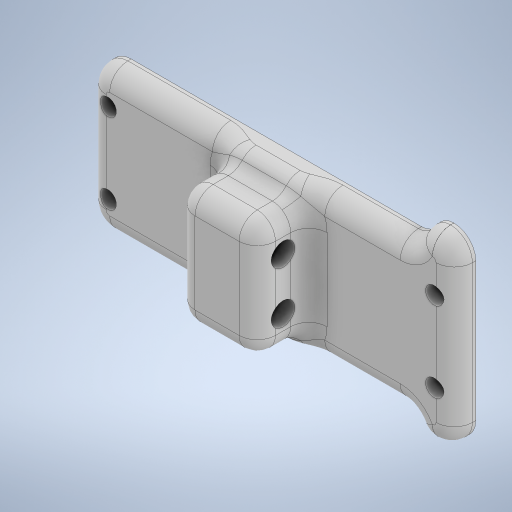
# Autodesk Inventor part: connecting plate servo flat v3
Saved by Autodesk Inventor 2024 (Build 280153000, 153)
## iProperties
Created: 2023-09-15
Part Number: connecting plate servo flat v3
Material: Generic
Document SubType Name: Modeling
Designer: chris
Density: 1 g/cm^3
Appearance: Default
Author: chris
Autodesk Inventor part; units mm, degrees
ref_plane "YZ Plane" through (0, 0, 0) normal (1, 0, 0) x (0, 1, 0)
ref_plane "XZ Plane" through (0, 0, 0) normal (0, 1, 0) x (-1, 0, 0)
ref_plane "XY Plane" through (0, 0, 0) normal (0, 0, 1) x (1, 0, 0)
sketch "Sketch1" plane through (0, 0, 0) normal (0, 0, 1) x (1, 0, 0)
  circle A0 centre (-10.2325, -6.35) radius 2
  circle A1 centre (-10.2325, 6.35) radius 2
  circle A2 centre (10.0875, 6.35) radius 2
  circle A3 centre (10.0875, -6.35) radius 2
  line L0 (-15.3125, 10.2775) -> (10.2325, 10.2775)
  line L1 (10.2325, 10.2775) -> (15.3125, 10.2775)
  line L2 (15.3125, 10.2775) -> (15.3125, -10.2775)
  line L3 (-15.3125, 10.2775) -> (-15.3125, -10.2775)
  line L4 (-15.3125, -10.2775) -> (15.3125, -10.2775)
  line L5 (0, -10.2775) -> (0, 10.2775)
  line L6 (-15.3125, 0) -> (0, 0)
  point P0 (0, 0)
  dimension "d1" = 5.08
  constraints: 14 end point, 4 centre point, 4 perpendicular, 3 midpoint, 1 point on line
  measures "d1" distance of L0.end L1.end
extrude "Extrusion1" add sketch "Sketch1" along normal blind 3.81 contours A0 | A1 | A2 | A3 | L0 L5 L6 L3 | L0 L1 L2 L4 L5 | L6 L5 L4 L3
sketch "Sketch2" plane through (0, 0, 3.81) normal (0, 0, 1) x (1, 0, 0)
  line L0 (-15.3125, -10.2775) -> (15.3125, -10.2775) projected
  line L1 (15.3125, -10.2775) -> (15.3125, 10.2775) projected
  line L2 (15.3125, 10.2775) -> (-15.3125, 10.2775) projected
  line L3 (-15.3125, 10.2775) -> (-15.3125, -10.2775) projected
  point P0 (0, 0)
extrude "Extrusion2" add sketch "Sketch2" along normal blind 1.5875
sketch "Sketch3" plane through (0, 0, 5.3975) normal (0, 0, 1) x (1, 0, 0)
  circle A0 centre (-10.2325, -6.35) radius 2 projected
  circle A1 centre (10.0875, -6.35) radius 2 projected
  circle A2 centre (10.0875, 6.35) radius 2 projected
  circle A3 centre (-10.2325, 6.35) radius 2 projected
  line L0 (-15.3125, -10.2775) -> (15.3125, -10.2775) projected
  line L1 (10.0875, -10.2775) -> (10.0875, 10.2775)
  line L2 (15.3125, 10.2775) -> (-15.3125, 10.2775) projected
  line L3 (-10.2325, -10.2775) -> (-10.2325, 10.2775)
  line L4 (-10.2325, 10.2775) -> (10.0875, 10.2775)
  line L5 (10.0875, -10.2775) -> (-10.2325, -10.2775)
  line L6 (15.3125, -10.2775) -> (15.3125, 10.2775) projected
  point P0 (0, 0)
  constraints: 8 end point, 2 point on line, 2 vertical, 1 parallel, 1 perpendicular
extrude "Extrusion3" add sketch "Sketch3" along normal blind 8.9916 contours A0 L3 | A0 L3 A3 L2 L1 A2 A1 L0 | L3 A3 | A1 L1 | L1 A2 picked at (-9.5825, -6.2017) picked at (-9.5825, 6.4983) picked at (9.4642, -6.5864) picked at (9.4642, 6.1136)
sketch "Sketch4" plane through (-10.2325, -10.2775, 5.3975) normal (-1, 0, 0) x (0, 0, 1)
  line L0 (8.9916, 20.555) -> (8.9916, 0) projected
  line L1 (8.9916, 10.2775) -> (0, 10.2775)
  line L2 (0, 0) -> (0, 20.555) projected
  line L3 (4.4958, 10.2775) -> (4.4958, 5.7817)
  line L4 (4.4958, 10.2775) -> (4.4958, 14.7733)
  circle A0 centre (4.4958, 5.7817) radius 2
  circle A1 centre (4.4958, 14.7733) radius 2
  point P0 (-5.3975, 10.2775)
  dimension "d8" = 4.4958
  dimension "d9" = 4.4958
  dimension "d10" = 4
  dimension "d11" = 4
  constraints: 6 end point, 3 midpoint, 2 centre point, 2 coincident, 2 vertical
  measures "d8" distance of L3.start L3.end
  measures "d9" distance of L3.start L4.end
  measures "d10" diameter of A0
  measures "d11" diameter of A1
extrude "Extrusion4" cut sketch "Sketch4" against normal through all
sketch "Sketch7" plane through (10.0875, -10.2775, 5.3975) normal (1, 0, 0) x (0, 0, -1)
  line L0 (0, 20.555) -> (0, 0) projected
  line L1 (0, 20.555) -> (-8.9916, 20.555) projected
  line L2 (-8.9916, 0) -> (-8.9916, 20.555) projected
  line L3 (0, 0) -> (-8.9916, 0) projected
  circle A0 centre (-4.4958, 14.7733) radius 2 projected
  circle A1 centre (-4.4958, 5.7817) radius 2 projected
  point P0 (5.3975, 10.2775)
extrude "Extrusion7" cut sketch "Sketch7" against normal blind 6.289 contours L0 L3 L2 L1 | A0 | A1
fillet "Fillet5" radius 3.175 8 edges at (-15.3125, 10.2775, 2.6987) (-15.3125, -10.2775, 2.6987) (15.3125, 10.2775, 2.6987) (15.3125, -10.2775, 2.6987) (3.7984, 10.2775, 9.8933) (-10.2325, 10.2775, 9.8933) (3.7984, -10.2775, 9.8933) (-10.2325, -10.2775, 9.8933)
sketch "Sketch9" plane through (0, 0, 0) normal (0, 0, -1) x (-1, 0, 0)
  line L0 (-34.8064, -15.875) -> (-34.8064, 15.875)
  line L1 (-27.8064, -15.875) -> (-34.8064, -15.875)
  line L2 (-27.8064, -12.5) -> (-27.8064, -15.875)
  line L3 (-27.8064, 12.5) -> (-27.8064, -12.5)
  line L4 (-27.8064, 15.875) -> (-27.8064, 12.5)
  line L5 (-34.8064, 15.875) -> (-27.8064, 15.875)
  line L6 (-27.8064, 12.5) -> (-27.8064, -12.5)
  line L7 (-27.8064, -12.5) -> (27.1936, -12.5)
  line L8 (27.1936, 12.5) -> (27.1936, -12.5)
  line L9 (27.1936, 12.5) -> (-27.8064, 12.5)
  line L10 (-34.8064, 0) -> (-27.8064, 0)
  line L11 (-31.3064, 0) -> (-31.3064, -6.985)
  line L12 (-31.3064, 0) -> (-31.3064, 6.985)
  circle A0 centre (-31.3064, -6.985) radius 1.5
  circle A1 centre (-31.3064, 6.985) radius 1.5
  circle A2 centre (23.6936, -6.985) radius 1.5
  circle A3 centre (23.6936, 6.985) radius 1.5
  line L13 (-34.8064, 0) -> (27.1936, 0)
  line L14 (0, 0) -> (0, 12.5)
  point P0 (0, 0)
  point P1 (-34.8064, 0)
  point P2 (-34.8064, 0)
  dimension "d26" = 6.985
  dimension "d27" = 6.985
  dimension "d28" = 3
  dimension "d29" = 3
  constraints: 30 end point, 4 centre point, 2 coincident, 2 midpoint, 2 point on line
  measures "d26" distance of L11.start L11.end
  measures "d27" distance of L11.start L12.end
  measures "d28" diameter of A0
  measures "d29" diameter of A1
extrude "Extrusion9" cut sketch "Sketch9" against normal up to surface (5.3975 mm away) contours L3 L13 L8 L7 | L3 L9 L14 L13 | L14 L9 L8 L13
sketch "Sketch10" plane through (0.6234, 10.2775, 5.3975) normal (0, 0, -1) x (-1, 0, 0)
  line L0 (10.856, -12.7733) -> (10.856, -16.7733) projected
  line L1 (10.856, -3.7817) -> (10.856, -7.7817) projected
  arc A0 (0, 0) -> (-3.175, -3.175) centre (0, -3.175) ccw projected
  arc A1 (0, 0) -> (-3.175, -3.175) centre (0, -3.175) ccw projected
  arc A2 (0, 0) -> (-3.175, -3.175) centre (0, -3.175) ccw projected
  arc A3 (0, 0) -> (-3.175, -3.175) centre (0, -3.175) ccw projected
  arc A4 (10.856, -3.175) -> (7.681, 0) centre (7.681, -3.175) ccw projected
  arc A5 (10.856, -3.175) -> (7.681, 0) centre (7.681, -3.175) ccw projected
  arc A6 (10.856, -3.175) -> (7.681, 0) centre (7.681, -3.175) ccw projected
  line L2 (-3.175, -3.7817) -> (-3.175, -7.7817) projected
  line L3 (-3.175, -3.7817) -> (-3.175, -7.7817) projected
  line L4 (10.856, -3.7817) -> (10.856, -7.7817) projected
  line L5 (-3.175, -12.7733) -> (-3.175, -16.7733) projected
  line L6 (-3.175, -17.38) -> (-3.175, -3.175) projected
  line L7 (-3.175, -3.175) -> (-3.175, -17.38) projected
  line L8 (-3.175, -17.38) -> (-3.175, -3.175) projected
  line L9 (-3.175, -3.7817) -> (-3.175, -7.7817) projected
  line L10 (-3.175, -12.7733) -> (-3.175, -16.7733) projected
  line L11 (-3.175, -3.175) -> (-3.175, -17.38) projected
  line L12 (10.856, -3.175) -> (10.856, -17.38) projected
  line L13 (10.856, -17.38) -> (10.856, -3.175) projected
  line L14 (10.856, -3.175) -> (10.856, -17.38) projected
  line L15 (10.856, -17.38) -> (10.856, -3.175) projected
  line L16 (10.856, -3.7817) -> (10.856, -7.7817) projected
  line L17 (10.856, -12.7733) -> (10.856, -16.7733) projected
  line L18 (-3.175, -12.7733) -> (-3.175, -16.7733) projected
  line L19 (10.856, -12.7733) -> (10.856, -16.7733) projected
  line L20 (7.681, -20.555) -> (0, -20.555) projected
  line L21 (7.681, -20.555) -> (0, -20.555) projected
  line L22 (7.681, -20.555) -> (0, -20.555) projected
  line L23 (7.681, -20.555) -> (0, -20.555) projected
  arc A7 (-3.175, -17.38) -> (0, -20.555) centre (0, -17.38) ccw projected
  arc A8 (-3.175, -17.38) -> (0, -20.555) centre (0, -17.38) ccw projected
  arc A9 (-3.175, -17.38) -> (0, -20.555) centre (0, -17.38) ccw projected
  arc A10 (7.681, -20.555) -> (10.856, -17.38) centre (7.681, -17.38) ccw projected
  arc A11 (7.681, -20.555) -> (10.856, -17.38) centre (7.681, -17.38) ccw projected
  line L24 (0, 0) -> (7.681, 0) projected
  arc A12 (0, 0) -> (-3.175, -3.175) centre (0, -3.175) ccw projected
  line L25 (-3.175, -3.175) -> (-3.175, -17.38) projected
  arc A13 (-3.175, -17.38) -> (0, -20.555) centre (0, -17.38) ccw projected
  line L26 (7.681, -20.555) -> (0, -20.555) projected
  arc A14 (7.681, -20.555) -> (10.856, -17.38) centre (7.681, -17.38) ccw projected
  line L27 (10.856, -17.38) -> (10.856, -3.175) projected
  arc A15 (10.856, -3.175) -> (7.681, 0) centre (7.681, -3.175) ccw projected
  arc A16 (-3.175, -17.38) -> (0, -20.555) centre (0, -17.38) ccw projected
  arc A17 (7.681, -20.555) -> (10.856, -17.38) centre (7.681, -17.38) ccw projected
  arc A18 (7.681, -20.555) -> (10.856, -17.38) centre (7.681, -17.38) ccw projected
  line L28 (7.681, -20.555) -> (0, -20.555) projected
  arc A19 (-3.175, -17.38) -> (0, -20.555) centre (0, -17.38) ccw projected
  line L29 (-3.175, -17.38) -> (-3.175, -3.175) projected
  arc A20 (0, 0) -> (-3.175, -3.175) centre (0, -3.175) ccw projected
  line L30 (0, 0) -> (7.681, 0) projected
  arc A21 (10.856, -3.175) -> (7.681, 0) centre (7.681, -3.175) ccw projected
  line L31 (10.856, -3.175) -> (10.856, -17.38) projected
  line L32 (0, 0) -> (7.681, 0) projected
  line L33 (0, 0) -> (7.681, 0) projected
  line L34 (0, 0) -> (7.681, 0) projected
  line L35 (0, 0) -> (7.681, 0) projected
  arc A22 (10.856, -3.175) -> (7.681, 0) centre (7.681, -3.175) ccw projected
  arc A23 (7.681, -20.555) -> (10.856, -17.38) centre (7.681, -17.38) ccw projected
  line L36 (0.6234, -10.2775) -> (0.6234, 2.2225) projected
  line L37 (0.6234, -10.2775) -> (-1.4597, -6.785)
  line L38 (8.1734, -10.2775) -> (-23.133, -10.2775)
  line L39 (-21.538, 5.5975) -> (-21.538, -26.1525)
  line L40 (-21.538, -26.1525) -> (-28.538, -26.1525)
  line L41 (-28.538, -26.1525) -> (-28.538, 5.5975)
  line L42 (-21.538, 5.5975) -> (-28.538, 5.5975)
  circle A24 centre (-25.038, -3.2925) radius 1.5
  circle A25 centre (-25.038, -17.2625) radius 1.5
  line L43 (-25.038, -10.2775) -> (-25.038, -17.2625)
  line L44 (-23.133, -10.2775) -> (-25.038, -10.2775)
  line L45 (-27.133, -22.7775) -> (-29.038, -22.7775)
  line L46 (-27.133, 2.2225) -> (-29.038, 2.2225)
  line L47 (0.6234, -10.2775) -> (2.7066, -13.77)
  line L48 (-21.538, -22.7775) -> (35.367, -22.7775)
  line L49 (35.367, -22.7775) -> (35.367, 2.2225)
  line L50 (35.367, 2.2225) -> (-21.538, 2.2225)
  circle A26 centre (31.867, -17.2625) radius 1.5
  circle A27 centre (31.867, -3.2925) radius 1.5
  line L51 (0.6234, -10.2775) -> (8.1734, -10.2775)
  point P0 (0.6234, -10.2775)
  point P1 (0.6234, -10.2775)
  point P2 (0, 0)
  dimension "d47" = 1.905
  dimension "d48" = 7.55
  constraints: 30 end point, 4 centre point, 2 point on line, 1 horizontal, 1 perpendicular, 11 other
  measures "d47" distance of L38.end L44.end
  measures "d48" distance of L36.start L51.end
extrude "Extrusion10" add sketch "Sketch10" along normal blind 3.75
fillet "Fillet17" radius 3.81 4 edges at (29.1614, -15.875, 3.5225) (-34.7436, -12.5, 3.5225) (-34.7436, 12.5, 3.5225) (29.1614, 15.875, 3.5225)
fillet "Fillet18" radius 3.175 2 edges at (22.1614, -15.875, 3.5225) (22.1614, 15.875, 3.5225)
fillet "Fillet19" radius 3.175 2 edges at (22.1614, -12.5, 3.5225) (22.1614, 12.5, 3.5225)
fillet "Fillet21" radius 3.175 16 edges at (-9.3026, 9.3476, 5.3975) (-10.2325, 0, 5.3975) (-9.3026, -9.3476, 5.3975) (-3.217, -10.2775, 5.3975) (2.8685, -9.3476, 5.3975) (3.7984, 0, 5.3975) (2.8685, 9.3476, 5.3975) (-3.217, 10.2775, 5.3975) (3.7984, 0, 14.3891) (2.8685, -9.3476, 14.3891) (-3.217, -10.2775, 14.3891) (-9.3026, -9.3476, 14.3891) (-10.2325, 0, 14.3891) (-9.3026, 9.3476, 14.3891) (-3.217, 10.2775, 14.3891) (2.8685, 9.3476, 14.3891)
fillet "Fillet22" radius 3.175 22 edges at (2.2985, 12.5, 5.4753) (-8.7326, 12.5, 5.4753) (-3.217, 12.5, 5.5437) (11.8475, 12.5, 5.3975) (21.3632, 12.9544, 5.3975) (23.6997, 15.4206, 5.3975) (25.3439, 15.875, 5.3975) (28.0455, 14.7591, 5.3975) (29.1614, 0, 5.3975) (28.0455, -14.7591, 5.3975) (25.3439, -15.875, 5.3975) (23.6997, -15.4206, 5.3975) (21.3632, -12.9544, 5.3975) (11.8475, -12.5, 5.3975) (2.2985, -12.5, 5.4753) (-8.7326, -12.5, 5.4753) (-3.217, -12.5, 5.5437) (-20.6681, -12.5, 5.3975) (-33.6277, -11.3841, 5.3975) (-34.7436, 0, 5.3975) (-33.6277, 11.3841, 5.3975) (-20.6681, 12.5, 5.3975)
body "Solid1"
